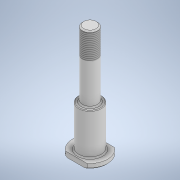
# Autodesk Inventor part: 62. Ось рычага управления
Saved by Autodesk Inventor 2021 (Build 250183000, 183)
## iProperties
Created: 2021-03-10
Part Number: 62. Ось рычага управления
Material: Типовые
Document SubType Name: Modeling
Designer: Данил
Density: 1 g/cm^3
Appearance: По умолчанию
Author: Данил
Autodesk Inventor part; units mm, degrees
ref_plane "YZ Plane" through (0, 0, 0) normal (1, 0, 0) x (0, 1, 0)
ref_plane "XZ Plane" through (0, 0, 0) normal (0, 1, 0) x (-1, 0, 0)
ref_plane "XY Plane" through (0, 0, 0) normal (0, 0, 1) x (1, 0, 0)
sketch "Эскиз1" plane through (0, 0, 0) normal (0, 0, 1) x (1, 0, 0)
  line L0 (0, 45) -> (0, -45)
  line L1 (0, -45) -> (13, -45)
  line L2 (14, -44) -> (14, -41)
  line L3 (14, -41) -> (10, -41)
  line L4 (9, -40) -> (9, -8.5)
  line L5 (8.5, -8) -> (7, -8)
  line L6 (6, -7) -> (6, 44)
  line L7 (5, 45) -> (0, 45)
  line L8 (14, -44) -> (13, -45)
  arc A0 (9, -40) -> (10, -41) centre (10, -40) ccw
  line L9 (9, -8.5) -> (8.5, -8)
  arc A1 (6, -7) -> (7, -8) centre (7, -7) ccw
  line L10 (6, 44) -> (5, 45)
  point P0 (0, 0)
  point P1 (0, 0)
  point P2 (14, -45)
  point P3 (9, -8)
  point P4 (6, 45)
  dimension "d0" = 90
  dimension "d1" = 28
  dimension "d2" = 1
  dimension "d3" = 45
  dimension "d4" = 4
  dimension "d5" = 1
  dimension "d6" = 18
  dimension "d7" = 0.5
  dimension "d8" = 45
  dimension "d9" = 1
  dimension "d10" = 12
  dimension "d11" = 33
  dimension "d12" = 1
  dimension "d13" = 45
  constraints: 22 end point, 6 perpendicular, 6 point on line, 4 point on circle, 4 tangent, 2 centre point, 1 coincident, 1 horizontal, 1 midpoint, 1 vertical
  measures "d0" distance of L0.start L0.end
  measures "d1" diameter of L2 L0
  measures "d2" distance of L2.start point (14, -45)
  measures "d3" angle of L2 L8
  measures "d4" distance between parallel lines of L1 L3
  measures "d5" radius of A0
  measures "d6" diameter of L4 L0
  measures "d7" distance of L4.end point (9, -8)
  measures "d8" angle of L4 L9
  measures "d9" radius of A1
  measures "d10" diameter of L6 L0
  measures "d11" distance between parallel lines of L5 L3
  measures "d12" distance of L6.end point (6, 45)
  measures "d13" angle of L6 L10
revolve "Вращение1" add sketch "Эскиз1" angle 360 about axis through (0, 45, 0) along (0, -1, 0)
sketch "Эскиз2" plane through (0, -45, 0) normal (0, -1, 0) x (1, 0, 0)
  line L0 (0, 11) -> (0, -11) construction
  line L1 (-14, 14) -> (14, 14)
  line L2 (14, 14) -> (14, 11)
  line L3 (14, 11) -> (-14, 11)
  line L4 (-14, 11) -> (-14, 14)
  circle A0 centre (0, 0) radius 14 projected
  point P0 (0, 0)
  point P1 (0, 0)
  dimension "d15" = 22
  dimension "d16" = 28
  constraints: 10 end point, 2 midpoint, 2 parallel, 1 coincident, 1 horizontal, 1 perpendicular, 1 tangent, 1 vertical
  measures "d15" distance of L0.start L0.end
  measures "d16" distance of L1.start L1.end
extrude "Выдавливание1" cut sketch "Эскиз2" against normal through all contours L1 A0 L3 L4 | L1 L2 L3 A0 | A0 L3 picked at (2.0072, 11.5463)
mirror "Зеркальное отражение1" about plane through (0, 0, 0) normal (0, 0, 1) of "Выдавливание1"
thread "Резьба1" size "M12x1.25" class "6g" standard "ISO Metric profile" length 20
